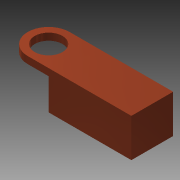
# Autodesk Inventor part: termination_lv_conductor
Saved by Autodesk Inventor 2014 SP1 (Build 180222100, 222)
## iProperties
Created: 2016-09-08
Part Number: termination_lv_conductor
Material: Copper, Cast
Document SubType Name: Modeling
Designer: tguillod
Density: 8.94 g/cm^3
Appearance: Copper - Satin
Author: tguillod
Autodesk Inventor part; units mm, degrees
ref_plane "YZ Plane" through (0, 0, 0) normal (1, 0, 0) x (0, 1, 0)
ref_plane "XZ Plane" through (0, 0, 0) normal (0, 1, 0) x (-1, 0, 0)
ref_plane "XY Plane" through (0, 0, 0) normal (0, 0, 1) x (1, 0, 0)
sketch "Sketch1" plane through (0, 0, 0) normal (0, 0, 1) x (1, 0, 0)
  line L0 (0, 0) -> (35.75, 0)
  line L1 (35.75, 0) -> (35.75, 12)
  line L2 (35.75, 12) -> (0, 12)
  line L3 (0, 12) -> (0, 0)
  dimension "d0" = 35.75
  dimension "d1" = 12
  constraints: 8 end point, 2 parallel, 1 horizontal, 1 perpendicular
  measures "d0" distance of L1.end L2.end
  measures "d1" distance of L0.end L1.end
extrude "Extrusion1" add sketch "Sketch1" along normal blind 11
sketch "Sketch5" plane through (0, 0, 0) normal (0, 0, -1) x (-1, 0, 0)
  line L0 (0, 12) -> (0, 0) projected
  line L1 (-35.75, 0) -> (-35.75, 12) projected
  line L2 (0, 0) -> (-35.75, 0) projected
  line L3 (-35.75, 12) -> (0, 12) projected
  line L4 (-35.75, 6) -> (0, 6) construction
  line L5 (-30.75, 12) -> (-30.75, 0) construction
  line L6 (-23.75, 12) -> (-23.75, 0) construction
  line L7 (-16.75, 12) -> (-16.75, 0) construction
  point P0 (-30.75, 6)
  point P1 (-23.75, 6)
  point P2 (-16.75, 6)
  dimension "d46" = 6
  dimension "d48" = 5
  dimension "d49" = 7
  dimension "d50" = 7
  constraints: 9 point on line, 8 end point, 5 midpoint, 4 perpendicular
  measures "d46" distance between parallel lines of L3 L4
  measures "d48" distance between parallel lines of L1 L5
  measures "d49" distance between parallel lines of L6 L5
  measures "d50" distance between parallel lines of L7 L6
hole "Hole3" at (30.75, 6, 0) at (23.75, 6, 0) at (16.75, 6, 0) direction (0, 0, 1) diameter 2.459 depth 8 tip angle 118 thread size "M3x0.5" class "6H" standard "ANSI Metric M Profile"
sketch "Sketch6" plane through (0, 0, 0) normal (0, 0, -1) x (-1, 0, 0)
  line L0 (0, 12) -> (0, 0) projected
  line L1 (-35.75, 0) -> (-35.75, 12) projected
  line L2 (0, 6) -> (-35.75, 6) construction
  point P0 (-6, 6)
  dimension "d35" = 6
  constraints: 2 end point, 2 midpoint, 1 point on line
  measures "d35" distance from line of L0 point (-6, 6)
hole "Hole4" at (6, 6, 0) direction (0, 0, 1) diameter 8 end through all
sketch "Sketch7" plane through (0, 0, 0) normal (0, 0, -1) x (-1, 0, 0)
  circle A0 centre (-6, 6) radius 4 projected
  line L0 (0, 0) -> (-35.75, 0) projected
  line L1 (0, 12) -> (-12, 12)
  line L2 (-12, 12) -> (-12, 0)
  line L3 (-12, 0) -> (0, 0)
  line L4 (0, 0) -> (0, 12)
  dimension "d43" = 12
  constraints: 8 end point, 2 parallel, 1 horizontal, 1 perpendicular, 1 point on line
  measures "d43" distance of L1.start L1.end
extrude "Extrusion3" cut sketch "Sketch7" against normal blind 9
fillet "Fillet5" radius 6 2 edges at (0, 12, 10) (0, 0, 10)
body "Solid1"
